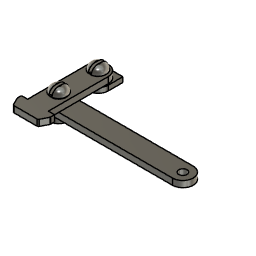
Servo Parallel Linkage v9 (Autodesk Fusion 360 design; units mm, degrees)
Autodesk Fusion 360 part; units mm, degrees
sketch "Sketch1" plane through (0, 0, 0) normal (0, 0, 1) x (1, 0, 0)
  line L0 (-15, 2.5) -> (15, 2.5)
  line L1 (15, -2.5) -> (-15, -2.5)
  arc A0 (-15, 2.5) -> (-15.0001, 2.5) centre (-15, 0) ccw
  arc A1 (-15.0001, 2.5) -> (-15, -2.5) centre (-15, 0) ccw
  arc A2 (17.3302, -0.9057) -> (15, 2.5) centre (15, 0) ccw
  arc A3 (15, -2.5) -> (17.3302, -0.9057) centre (15, 0) ccw
  circle A4 centre (-15, 0) radius 1.75
  circle A5 centre (15, 0) radius 0.5
  line L2 (0, 0) -> (0, -2.5)
  line L3 (0, 0) -> (0, 2.5)
  dimension "d3" = 2.5
  dimension "d4" = 2.5
  dimension "d5" = 3.5
  dimension "d6" = 1
  dimension "d88" = 5
  dimension "d89" = 30
  constraint horizontal L0
  constraint parallel L0 L1
  constraint coincident L2.start L3.start
  constraint tangent L0 A0
  constraint tangent L1 A1
  constraint coincident A0.end A1.start
  constraint tangent L0 A2
  constraint equal A1 A2
  constraint tangent L1 A3
  constraint equal A1 A3
  constraint coincident A2.start A3.end
  constraint midpoint L1 L2.end
  constraint midpoint L0 L3.end
  constraint equal L2 L3
  constraint perpendicular L1 L2
  constraint perpendicular L0 L3
  constraint coincident A0.centre A1.centre
  constraint coincident A2.centre A3.centre
  constraint equal L0 L1
  measures "d3" radius of A0
  measures "d4" radius of A1
  measures "d5" diameter of A4
  measures "d6" diameter of A5
  measures "d88" distance of L0 L1
  measures "d89" distance of L0.start L0.end
extrude "Extrude1" add sketch "Sketch1" along normal blind 1.5 makes body 1
sketch "Sketch2" plane through (0, 0, 1.5) normal (0, 0, 1) x (-1, 0, 0)
  circle A0 centre (-15, 0) radius 0.5
  circle A1 centre (15, 0) radius 1.75
  arc A2 (15, -2.5) -> (15, 2.5) centre (15, 0) ccw
  line L0 (15, 2.5) -> (-15, 2.5)
  arc A3 (-15, 2.5) -> (-15, -2.5) centre (-15, 0) ccw
  line L1 (-15, -2.5) -> (15, -2.5)
  circle A4 centre (11.5, 0) radius 1.75
  line L2 (9, -9.5) -> (9, 5)
  line L3 (14, 5) -> (14, -9.5)
  line L4 (11.5, 5) -> (7.5, 5)
  line L5 (11.5, 5) -> (15.5, 5)
  line L6 (7.5, 5) -> (7.5, 5.941)
  line L7 (11.5, 8) -> (14.2775, 8)
  line L8 (11.5, 8) -> (8.7225, 8)
  line L9 (8.4005, 7.801) -> (7.5264, 6.0528)
  line L10 (15.5, 5) -> (15.5, 5.941)
  line L11 (15.4736, 6.0528) -> (14.5995, 7.801)
  arc A5 (8.7225, 8) -> (8.4005, 7.801) centre (8.7225, 7.64) ccw
  arc A6 (14.5995, 7.801) -> (14.2775, 8) centre (14.2775, 7.64) ccw
  arc A7 (7.5264, 6.0528) -> (7.5, 5.941) centre (7.75, 5.941) ccw
  arc A8 (15.5, 5.941) -> (15.4736, 6.0528) centre (15.25, 5.941) ccw
  line L12 (14, 0) -> (13.25, 0)
  line L13 (9, 5) -> (7.5, 5)
  line L14 (14, 5) -> (15.5, 5)
  line L15 (9.75, 0) -> (9, 0)
  arc A9 (9, -9.5) -> (11.5, -12) centre (11.5, -9.5) ccw
  arc A10 (11.5, -12) -> (14, -9.5) centre (11.5, -9.5) ccw
  circle A11 centre (11.5, -9.5) radius 1.75
  point P0 (11.5, 0)
  point P1 (11.5, 0)
  point P2 (11.5, 0)
  point P3 (14, -12)
  point P4 (7.5, 6)
  point P5 (14.5, 8)
  point P6 (8.5, 8)
  point P7 (15.5, 6)
  dimension "d62" = 3.5
  dimension "d65" = 4
  dimension "d66" = 4
  dimension "d67" = 5
  dimension "d73" = 3
  dimension "d75" = 1
  dimension "d76" = 3
  dimension "d77" = 3
  dimension "d78" = 1
  dimension "d79" = 0.36
  dimension "d80" = 0.36
  dimension "d81" = 0.25
  dimension "d82" = 0.25
  dimension "d83" = 5
  dimension "d84" = 12
  dimension "d85" = 2.5
  dimension "d86" = 2.5
  dimension "d87" = 3.5
  constraint coincident A1.centre P1
  constraint coincident P2 P1
  constraint concentric A1 A4
  constraint parallel L2 L3
  constraint horizontal L4
  constraint perpendicular L3 L5
  constraint coincident L5 L3.start
  constraint coincident L4 L2.end
  constraint perpendicular L4 L6
  constraint horizontal L7
  constraint horizontal L8
  constraint perpendicular L5 L10
  constraint coincident P6 L8
  constraint coincident P6 L9
  constraint tangent L8 A5
  constraint tangent L9 A5
  constraint coincident P5 L7
  constraint coincident P5 L11
  constraint tangent L7 A6
  constraint tangent L11 A6
  constraint coincident P4 L6
  constraint coincident P4 L9
  constraint tangent L6 A7
  constraint tangent L9 A7
  constraint coincident P7 L10
  constraint coincident P7 L11
  constraint tangent L10 A8
  constraint tangent L11 A8
  constraint coincident A4 L12.end
  constraint perpendicular L2 L4
  constraint coincident L3 L12.start
  constraint perpendicular L3 L12
  constraint coincident A4 L15.start
  constraint coincident L2 L15.end
  constraint perpendicular L2 L15
  constraint equal L12 L15
  constraint equal L6 L10
  constraint tangent L2 A9
  constraint coincident L3 P3
  constraint tangent L3 A10
  constraint coincident A9.end A10.start
  constraint concentric A10 A11
  measures "d62" diameter of A4
  measures "d65" distance of L4.start L4.end
  measures "d66" distance of L4.start L5.end
  measures "d67" distance of P2 L5
  measures "d73" distance of L4.start L7.start
  measures "d75" distance of L4.end P4
  measures "d76" distance of L7.start P5
  measures "d77" distance of L7.start P6
  measures "d78" distance of L5.end P7
  measures "d79" radius of A5
  measures "d80" radius of A6
  measures "d81" radius of A7
  measures "d82" radius of A8
  measures "d83" distance of L2 L3
  measures "d84" distance of P3 L12.start
  measures "d85" radius of A9
  measures "d86" radius of A10
  measures "d87" diameter of A11
extrude "Extrude2" add sketch "Sketch2" along normal blind 1.5 separate body contours A1 L3 L12 | A1 L0 A4 L2 L3 L15 | A1 L1 A4 L2 L3 L15 | A1 L3 L12 | L0 L2 L3 L4 L5 | L1 L2 L3 A9 A10 | L4 L5 L6 L7 L8 L9 L10 L11 A5 A6 A7 A8 L13 L14 makes body 2
sketch "Sketch4" plane through (0, 0, 0) normal (0, 0, 1) x (1, 0, 0)
  circle A0 centre (-11.5, 11) radius 1.5
  circle A1 centre (-11.5, 11) radius 2
  line L0 (-13.5002, 11.0293) -> (-13.5002, 13.0293)
  line L1 (-13.5002, 13.0293) -> (-9.5002, 13.0293)
  line L2 (-9.5002, 13.0293) -> (-9.5002, 11.0293)
  line L3 (-13.4998, 11.0293) -> (-13.5002, 11.0293)
  dimension "d22" = 4
  dimension "d33" = 4
  dimension "d34" = 2
  constraint concentric A0 A1
  constraint vertical L0
  constraint horizontal L1
  constraint vertical L2
  constraint coincident A1 L2.end
  constraint coincident A1 L3.start
  measures "d22" diameter of A1
  measures "d33" distance of L2.end L0.start
  measures "d34" distance of L2.end L1.end
sketch "Sketch6" plane through (0, 0, 3) normal (0, 0, 1) x (-1, 0, 0)
  circle A0 centre (11.5, 0) radius 1.75
  line L0 (9, 5) -> (9, -9.5)
  line L1 (14, -9.5) -> (14, 5)
  line L2 (14, 5) -> (15.5, 5)
  circle A1 centre (11.5, -9.5) radius 1.75
  arc A2 (9, -9.5) -> (14, -9.5) centre (11.5, -9.5) ccw
  line L3 (15.5, 5) -> (15.5, 5.941)
  arc A3 (15.5, 5.941) -> (15.4736, 6.0528) centre (15.25, 5.941) ccw
  line L4 (15.4736, 6.0528) -> (14.5995, 7.801)
  arc A4 (14.5995, 7.801) -> (14.2775, 8) centre (14.2775, 7.64) ccw
  line L5 (14.2775, 8) -> (8.7225, 8)
  arc A5 (8.7225, 8) -> (8.4005, 7.801) centre (8.7225, 7.64) ccw
  line L6 (8.4005, 7.801) -> (7.5264, 6.0528)
  arc A6 (7.5264, 6.0528) -> (7.5, 5.941) centre (7.75, 5.941) ccw
  line L7 (7.5, 5.941) -> (7.5, 5)
  line L8 (7.5, 5) -> (9, 5)
move_body "Move1" bodies 2 to x (1, 0, 0) y (0, 1, 0) z (0, 0, 1) at (-3.5, 0, 0)
move_face "OffsetFaces4" offset -0.5 1 faces at (14.6692, -0.3749, 1) on bodies 1
ref_plane "WorkPlane2" through (0, 0, -0.4) normal (0, 0, -1) x (-1, 0, 0)
sketch "Sketch7" plane through (0, 0, -0.4) normal (0, 0, -1) x (-1, 0, 0)
  circle A0 centre (15, 0) radius 2.5
  dimension "d92" = 5
  measures "d92" diameter of A0
extrude "Extrude6" add sketch "Sketch7" along normal blind 1.2 separate body makes body 3
sketch "Sketch8" plane through (0, 0, -0.4) normal (0, 0, 1) x (-1, 0, 0)
  circle A0 centre (15, 0) radius 2.5
  line L0 (15.35, 1.4586) -> (15.35, -1.4586)
  line L1 (14.65, -1.4586) -> (14.65, 1.4586)
  arc A1 (14.65, 1.4586) -> (14.65, -1.4586) centre (15, 0) ccw
  arc A2 (15.35, -1.4586) -> (15.35, 1.4586) centre (15, 0) ccw
  point P0 (15, 0)
  dimension "d95" = 3
  constraint concentric A0 A1
  constraint coincident P0 A0.centre
  constraint coincident L0.end A1
  constraint concentric A1 A2
  measures "d95" diameter of A1
extrude "Extrude7" add sketch "Sketch8" along normal blind 3.7 contours L0 A2 | L1 A1 bodies 3
ref_plane "WorkPlane3" through (-15.925, 0, 3.3) normal (0, 0, 1) x (-1, 0, 0)
sketch "Sketch9" plane through (0, 0, 3.3) normal (0, 0, 1) x (1, 0, 0)
  line L0 (-15.35, 1.9691) -> (-15.35, -1.9691)
  line L1 (-14.65, -1.9691) -> (-14.65, 1.9691)
  arc A0 (-14.65, -1.9691) -> (-14.65, 1.9691) centre (-15, 0) ccw
  arc A1 (-15.35, 1.9691) -> (-15.35, -1.9691) centre (-15, 0) ccw
  point P0 (-15, 0)
  dimension "d100" = 4
  constraint parallel L0 L1
  constraint coincident P0 A0.centre
  constraint coincident L0.start A0
  constraint concentric A0 A1
  measures "d100" diameter of A0
extrude "Extrude8" add sketch "Sketch9" along normal blind 1.5 bodies 3
fillet "Fillet3" radius 1.5 2 edges at (-13, 0, 4.8) (-17, 0, 4.8) on bodies 3
sketch "Sketch10" plane through (0, 0, 0) normal (0, 0, 1) x (1, 0, 0)
  circle A0 centre (-15, 0) radius 1.75
  line L0 (-17.5, 9.5) -> (-17.5, -5)
  line L1 (-17.5, -5) -> (-19, -5)
  line L2 (-19, -5) -> (-19, -5.941)
  arc A1 (-19, -5.941) -> (-18.9736, -6.0528) centre (-18.75, -5.941) ccw
  line L3 (-18.9736, -6.0528) -> (-18.0995, -7.801)
  arc A2 (-18.0995, -7.801) -> (-17.7775, -8) centre (-17.7775, -7.64) ccw
  line L4 (-17.7775, -8) -> (-12.2225, -8)
  arc A3 (-12.2225, -8) -> (-11.9005, -7.801) centre (-12.2225, -7.64) ccw
  line L5 (-11.9005, -7.801) -> (-11.0264, -6.0528)
  arc A4 (-11.0264, -6.0528) -> (-11, -5.941) centre (-11.25, -5.941) ccw
  line L6 (-11, -5.941) -> (-11, -5)
  line L7 (-11, -5) -> (-12.5, -5)
  line L8 (-12.5, -5) -> (-12.5, 9.5)
  line L9 (-14.65, -1.4586) -> (-14.65, 1.4586)
  arc A5 (-14.65, -1.4586) -> (-14.65, 1.4586) centre (-15, 0) ccw
  line L10 (-15.35, 1.4586) -> (-15.35, -1.4586)
  arc A6 (-15.35, 1.4586) -> (-15.35, -1.4586) centre (-15, 0) ccw
  circle A7 centre (-15, 0) radius 2.5
  line L11 (-17.5, 9.5) -> (-17.5, 13)
  line L12 (-17.5, 13) -> (-12.5, 13)
  line L13 (-12.5, 13) -> (-12.5, 9.5)
  arc A8 (-17.5, 9.5) -> (-12.5, 9.5) centre (-15, 9.5) ccw
  dimension "d106" = 5
  dimension "d107" = 3.5
  constraint vertical L11
  constraint horizontal L12
  constraint vertical L13
  constraint tangent L13 A8
  measures "d106" distance of L8.end L0.start
  measures "d107" distance of L8.end L12.end
extrude "Extrude9" add sketch "Sketch10" along normal blind 1.2 separate body contours L11 L12 L13 A8 makes body 4
sketch "Sketch11" plane through (0, 0, 1.2) normal (0, 0, 1) x (-1, 0, 0)
  line L0 (17.5, -13) -> (17.5, -9.5)
  arc A0 (17.5, -9.5) -> (12.5, -9.5) centre (15, -9.5) ccw
  line L1 (12.5, -9.5) -> (12.5, -13)
  line L2 (12.5, -13) -> (17.5, -13)
  line L3 (14.65, 1.4586) -> (14.65, -1.4586)
  arc A1 (14.65, 1.4586) -> (14.65, -1.4586) centre (15, 0) ccw
  line L4 (15.35, -1.4586) -> (15.35, 1.4586)
  arc A2 (15.35, -1.4586) -> (15.35, 1.4586) centre (15, 0) ccw
  circle A3 centre (15, 0) radius 2.5
  circle A4 centre (15, 0) radius 1.75
  circle A5 centre (15, -9.5) radius 1.75
  arc A6 (12.5, -9.5) -> (17.5, -9.5) centre (15, -9.5) ccw
  line L5 (17.5, -9.5) -> (17.5, 5)
  line L6 (17.5, 5) -> (19, 5)
  line L7 (19, 5) -> (19, 5.941)
  arc A7 (19, 5.941) -> (18.9736, 6.0528) centre (18.75, 5.941) ccw
  line L8 (18.9736, 6.0528) -> (18.0995, 7.801)
  arc A8 (18.0995, 7.801) -> (17.7775, 8) centre (17.7775, 7.64) ccw
  line L9 (17.7775, 8) -> (12.2225, 8)
  arc A9 (12.2225, 8) -> (11.9005, 7.801) centre (12.2225, 7.64) ccw
  line L10 (11.9005, 7.801) -> (11.0264, 6.0528)
  arc A10 (11.0264, 6.0528) -> (11, 5.941) centre (11.25, 5.941) ccw
  line L11 (11, 5.941) -> (11, 5)
  line L12 (11, 5) -> (12.5, 5)
  line L13 (12.5, 5) -> (12.5, -9.5)
  line L14 (14.65, -8.0414) -> (14.65, -10.9586)
  line L15 (15.35, -8.0414) -> (15.35, -10.9586)
  arc A11 (14.65, -8.0414) -> (14.65, -10.9586) centre (15, -9.5) ccw
  arc A12 (15.35, -10.9586) -> (15.35, -8.0414) centre (15, -9.5) ccw
  dimension "d110" = 3
  constraint concentric A6 A11
  constraint vertical L14
  constraint coincident L15.end A11
  constraint parallel L14 L15
  constraint concentric A11 A12
  measures "d110" diameter of A11
extrude "Extrude10" add sketch "Sketch11" along normal blind 2 contours L14 A11 | L15 A12 bodies 4
ref_plane "WorkPlane4" through (-14.075, 9.5, 3.2) normal (0, 0, 1) x (-1, 0, 0)
sketch "Sketch12" plane through (0, 0, 3.2) normal (0, 0, 1) x (1, 0, 0)
  line L0 (-15.35, 10.9586) -> (-15.35, 8.0414)
  arc A0 (-15.35, 10.9586) -> (-15.35, 8.0414) centre (-15, 9.5) ccw
  line L1 (-14.65, 8.0414) -> (-14.65, 10.9586)
  arc A1 (-14.65, 8.0414) -> (-14.65, 10.9586) centre (-15, 9.5) ccw
  line L2 (-17.5, 13) -> (-17.5, 9.5)
  arc A2 (-17.5, 9.5) -> (-12.5, 9.5) centre (-15, 9.5) ccw
  line L3 (-12.5, 9.5) -> (-12.5, 13)
  line L4 (-12.5, 13) -> (-17.5, 13)
  circle A3 centre (-15, 9.5) radius 2
  line L5 (-14.65, 11.4691) -> (-14.65, 7.5309)
  line L6 (-15.35, 11.4691) -> (-15.35, 7.5309)
  dimension "d114" = 4
  constraint concentric A2 A3
  constraint coincident A3 L5.start
  constraint coincident A3 L5.end
  constraint parallel L1 L5
  constraint coincident A3 L6.start
  constraint coincident A3 L6.end
  constraint parallel L0 L6
  measures "d114" diameter of A3
extrude "Extrude11" add sketch "Sketch12" along normal blind 1.5 contours L0 A0 L6 | A0 A3 L6 | A1 A3 L5 | L1 A1 L5 bodies 4
fillet "Fillet4" radius 1.5 2 edges at (-13, 9.5, 4.7) (-17, 9.5, 4.7) on bodies 4
extrude "Extrude4" [suppressed]
sketch "Sketch3" plane through (0, 0, 1.5) normal (0, 0, 1) x (1, 0, 0)
  circle A0 centre (-11.5, 11) radius 1.5
  line L0 (-11.75, 9.7243) -> (-11.75, 12.2757)
  arc A1 (-11.25, 9.7243) -> (-11.25, 12.2757) centre (-11.5, 11) ccw
  arc A2 (-11.75, 12.2757) -> (-11.75, 9.7243) centre (-11.5, 11) ccw
  line L1 (-11.25, 12.2757) -> (-11.25, 9.7243)
  arc A3 (-13.4998, 11.0293) -> (-9.5002, 11.0293) centre (-11.5, 11) ccw
  line L2 (-9.5002, 11.0293) -> (-9.5002, 13.0293)
  line L3 (-9.5002, 13.0293) -> (-13.5002, 13.0293)
  line L4 (-13.5002, 13.0293) -> (-13.5002, 11.0293)
  line L5 (-13.5002, 11.0293) -> (-13.4998, 11.0293)
  point P0 (-11.5, 11)
  constraint coincident P0 A0.centre
  constraint concentric A0 A1
  constraint concentric A1 A2
extrude "Extrude3" [suppressed]
ref_plane "WorkPlane1" through (-11.5, 3.5941, 3.2) normal (0, 0, -1) x (1, 0, 0)
sketch "Sketch5" plane through (0, 0, 3.2) normal (0, 0, -1) x (-1, 0, 0)
  line L0 (11.75, 12.2757) -> (11.75, 9.7243)
  arc A0 (11.75, 9.7243) -> (11.75, 12.2757) centre (11.5, 11) ccw
  arc A1 (11.25, 12.2757) -> (11.25, 9.7243) centre (11.5, 11) ccw
  line L1 (11.25, 9.7243) -> (11.25, 12.2757)
  line L2 (11.25, 9.2679) -> (11.25, 12.7321)
  line L3 (11.75, 9.2679) -> (11.75, 12.7321)
  arc A2 (11.75, 9.2679) -> (11.75, 12.7321) centre (11.5, 11) ccw
  arc A3 (11.25, 12.7321) -> (11.25, 9.2679) centre (11.5, 11) ccw
  arc A4 (9.5002, 11.0293) -> (13.4998, 11.0293) centre (11.5, 11) ccw
  line L4 (9.5002, 11.0293) -> (9.5002, 13.0293)
  line L5 (9.5002, 13.0293) -> (13.5002, 13.0293)
  line L6 (13.5002, 13.0293) -> (13.5002, 11.0293)
  line L7 (13.5002, 11.0293) -> (13.4998, 11.0293)
  dimension "d26" = 3.5
  constraint concentric A0 A2
  constraint coincident L2.end A2
  constraint parallel L1 L2
  constraint parallel L0 L3
  constraint concentric A2 A3
  measures "d26" diameter of A2
extrude "Extrude5" [suppressed]
fillet "Fillet1" [suppressed]
fillet "Fillet2" [suppressed]
move_face "OffsetFaces1" [suppressed]
move_face "OffsetFaces2" [suppressed]
move_face "OffsetFaces3" [suppressed]
equation "d107 = 2.5 mm + 1 mm"
named bodies: "Top Part", "Pin Pusher", "Connector", "Pin Holder 1", "Pin Holder 2"
